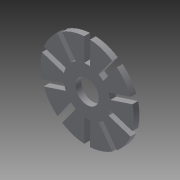
# Autodesk Inventor part: HeatSinkWasher
Saved by Autodesk Inventor 2014 SP1 (Build 180222100, 222)
## iProperties
Created: 2013-12-26
Part Number: HeatSinkWasher
Material: Generic
Document SubType Name: Modeling
Designer: Jack
Density: 1 g/cm^3
Appearance: Default
Author: Jack
Autodesk Inventor part; units mm, degrees
ref_plane "YZ Plane" through (0, 0, 0) normal (1, 0, 0) x (0, 1, 0)
ref_plane "XZ Plane" through (0, 0, 0) normal (0, 1, 0) x (-1, 0, 0)
ref_plane "XY Plane" through (0, 0, 0) normal (0, 0, 1) x (1, 0, 0)
sketch "Sketch1" plane through (0, 0, 0) normal (0, 1, 0) x (-1, 0, 0)
  line L0 (0, 6.4) -> (0.794, 6.4)
  line L1 (0, 6.4) -> (-0.794, 6.4)
  line L2 (0.794, 6.4) -> (0.794, 12.6752)
  line L3 (-0.794, 6.4) -> (-0.794, 12.6752)
  line L4 (3.7618, 5.1777) -> (4.4042, 4.711)
  line L5 (3.7618, 5.1777) -> (3.1195, 5.6444)
  line L6 (4.4042, 4.711) -> (8.0926, 9.7877)
  line L7 (3.1195, 5.6444) -> (6.8079, 10.7211)
  line L8 (6.0868, 1.9777) -> (6.3321, 1.2226)
  line L9 (6.0868, 1.9777) -> (5.8414, 2.7328)
  line L10 (6.3321, 1.2226) -> (12.3001, 3.1617)
  line L11 (5.8414, 2.7328) -> (11.8094, 4.672)
  line L12 (6.0868, -1.9777) -> (5.8414, -2.7328)
  line L13 (6.0868, -1.9777) -> (6.3321, -1.2226)
  line L14 (5.8414, -2.7328) -> (11.8094, -4.672)
  line L15 (6.3321, -1.2226) -> (12.3001, -3.1617)
  line L16 (3.7618, -5.1777) -> (3.1195, -5.6444)
  line L17 (3.7618, -5.1777) -> (4.4042, -4.711)
  line L18 (3.1195, -5.6444) -> (6.8079, -10.7211)
  line L19 (4.4042, -4.711) -> (8.0926, -9.7877)
  line L20 (0, -6.4) -> (-0.794, -6.4)
  line L21 (0, -6.4) -> (0.794, -6.4)
  line L22 (-0.794, -6.4) -> (-0.794, -12.6752)
  line L23 (0.794, -6.4) -> (0.794, -12.6752)
  line L24 (-3.7618, -5.1777) -> (-4.4042, -4.711)
  line L25 (-3.7618, -5.1777) -> (-3.1195, -5.6444)
  line L26 (-4.4042, -4.711) -> (-8.0926, -9.7877)
  line L27 (-3.1195, -5.6444) -> (-6.8079, -10.7211)
  line L28 (-6.0868, -1.9777) -> (-6.3321, -1.2226)
  line L29 (-6.0868, -1.9777) -> (-5.8414, -2.7328)
  line L30 (-6.3321, -1.2226) -> (-12.3001, -3.1617)
  line L31 (-5.8414, -2.7328) -> (-11.8094, -4.672)
  line L32 (-6.0868, 1.9777) -> (-5.8414, 2.7328)
  line L33 (-6.0868, 1.9777) -> (-6.3321, 1.2226)
  line L34 (-5.8414, 2.7328) -> (-11.8094, 4.672)
  line L35 (-6.3321, 1.2226) -> (-12.3001, 3.1617)
  line L36 (-3.7618, 5.1777) -> (-3.1195, 5.6444)
  line L37 (-3.7618, 5.1777) -> (-4.4042, 4.711)
  line L38 (-3.1195, 5.6444) -> (-6.8079, 10.7211)
  line L39 (-4.4042, 4.711) -> (-8.0926, 9.7877)
  arc A0 (6.8079, 10.7211) -> (0.794, 12.6752) centre (0, 0) ccw
  arc A1 (-0.794, 12.6752) -> (-6.8079, 10.7211) centre (0, 0) ccw
  arc A2 (-8.0926, 9.7877) -> (-11.8094, 4.672) centre (0, 0) ccw
  arc A3 (-12.3001, 3.1617) -> (-12.3001, -3.1617) centre (0, 0) ccw
  arc A4 (-11.8094, -4.672) -> (-8.0926, -9.7877) centre (0, 0) ccw
  arc A5 (-6.8079, -10.7211) -> (-0.794, -12.6752) centre (0, 0) ccw
  arc A6 (0.794, -12.6752) -> (6.8079, -10.7211) centre (0, 0) ccw
  arc A7 (8.0926, -9.7877) -> (11.8094, -4.672) centre (0, 0) ccw
  arc A8 (12.3001, -3.1617) -> (12.3001, 3.1617) centre (0, 0) ccw
  arc A9 (11.8094, 4.672) -> (8.0926, 9.7877) centre (0, 0) ccw
  circle A10 centre (0, 0) radius 3.175
  dimension "d1" = 0.794
  dimension "d2" = 0.794
  dimension "d3" = 6.4
  dimension "d6" = 360
  dimension "d8" = 12.7
  dimension "d9" = 6.35
  constraints: 80 end point, 20 point on circle, 11 centre point, 4 coincident, 2 equal length, 1 horizontal, 1 perpendicular, 1 vertical alignment, 98 other
  measures "d1" distance of L0.start L0.end
  measures "d2" distance of L0.start L1.end
  measures "d3" distance of point (0, 0) L0.start
  measures "d8" radius of A8
  measures "d9" diameter of A10
extrude "Extrusion1" add sketch "Sketch1" along normal blind 1.556
body "Solid1"
